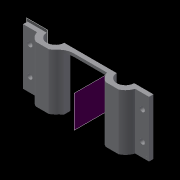
# Autodesk Inventor part: V2 GantryCover
Saved by Autodesk Inventor 2014 (Build 180170000, 170)
## iProperties
Created: 2015-07-08
Part Number: V2 GantryCover
Material: Generic
Document SubType Name: Modeling
Designer: Scott
Density: 1 g/cm^3
Appearance: Default
Author: Scott
Autodesk Inventor part; units mm, degrees
ref_plane "YZ Plane" through (0, 0, 0) normal (1, 0, 0) x (0, 1, 0)
ref_plane "XZ Plane" through (0, 0, 0) normal (0, 1, 0) x (-1, 0, 0)
ref_plane "XY Plane" through (0, 0, 0) normal (0, 0, 1) x (1, 0, 0)
ref_plane "Work Plane1" through (0, 0, 0) normal (0, 0, 1) x (1, 0, 0)
sketch "Sketch1" plane through (0, 0, 0) normal (0, 0, 1) x (1, 0, 0)
  line L0 (-85.1434, -2.54) -> (-85.1434, 45.54) projected
  circle A0 centre (-90.9267, 33.52) radius 2.2225 projected
  circle A1 centre (-90.9267, 9.48) radius 2.2225 projected
  line L1 (-80.2, 45.54) -> (-80.2, -2.54) projected
  line L2 (-80.2, 45.54) -> (-96.71, 45.54) projected
  line L3 (-96.71, 45.54) -> (-96.71, -2.54) projected
  line L4 (-96.71, -2.54) -> (-80.2, -2.54) projected
  line L5 (-20.2, 45.54) -> (-60, 45.54) projected
  circle A2 centre (5.5267, 9.48) radius 2.2225 projected
  circle A3 centre (5.5267, 33.52) radius 2.2225 projected
  line L6 (-5.2, -2.54) -> (-5.2, 45.54) projected
  line L7 (-5.2, -2.54) -> (11.31, -2.54) projected
  line L8 (11.31, 0) -> (11.31, -2.54) projected
  line L9 (11.31, 0) -> (0, 0) projected
  line L10 (0, 0.0064) -> (0, 0) projected
  line L11 (0, 0.0064) -> (11.31, 0.0064) projected
  line L12 (11.31, 0.0064) -> (11.31, 45.54) projected
  line L13 (11.31, 45.54) -> (-5.2, 45.54) projected
  line L14 (-25.4, 27.506) -> (-25.4, 43) projected
  line L15 (-25.4, 27.506) -> (-21.745, 27.506) projected
  line L16 (-21.745, 27.506) -> (-21.745, 3.376) projected
  line L17 (-21.745, 3.376) -> (-25.4, 3.376) projected
  line L18 (-25.4, -2.54) -> (-25.4, 3.376) projected
  line L19 (-25.4, -2.54) -> (-20.2, -2.54) projected
  line L20 (-20.2, 45.54) -> (-20.2, -2.54) projected
  line L21 (-20.2, 45.54) -> (-60, 45.54) projected
  line L22 (-60, 45.54) -> (-60, 43) projected
  line L23 (-60, 43) -> (-25.4, 43) projected
  line L24 (-65.2, -2.54) -> (-65.2, 45.54) projected
  line L25 (-65.2, -2.54) -> (-60, -2.54) projected
  line L26 (-60, 43) -> (-60, -2.54) projected
  line L27 (-60, 45.54) -> (-60, 43) projected
  line L28 (-60, 45.54) -> (-65.2, 45.54) projected
extrude "Extrusion1" add sketch "Sketch1" along normal blind 3.81
sketch "Sketch2" plane through (-96.71, 45.54, 0) normal (0, 1, 0) x (1, 0, 0)
  line L0 (0, 0) -> (16.51, 0) projected
  arc A0 (31.51, 0) -> (16.51, 0) centre (24.01, 0) ccw projected
  arc A1 (16.51, 0) -> (31.51, 0) centre (24.01, 0) ccw
  arc A2 (11.3049, 0) -> (36.7151, 0) centre (24.01, 0) ccw
  line L1 (16.51, 0) -> (11.3049, 0)
  line L2 (31.51, 0) -> (36.7151, 0)
  arc A3 (91.51, 0) -> (76.51, 0) centre (84.01, 0) ccw projected
  arc A4 (76.51, 0) -> (91.51, 0) centre (84.01, 0) ccw
  line L3 (96.71, 0) -> (91.51, 0)
  line L4 (76.51, 0) -> (71.31, 0)
  arc A5 (71.31, 0) -> (96.71, 0) centre (84.01, 0) ccw
  dimension "d3" = 12.7
  constraints: 8 end point, 8 point on circle, 4 centre point, 3 coincident, 3 collinear, 2 concentric, 1 point on line
  measures "d3" radius of A5
extrude "Extrusion2" add sketch "Sketch2" against normal up to surface (48.08 mm away) contours L0 A1 L2 A2 | L3 A5 L4 A4
ref_plane "Work Plane2" through (-42.7, 0, 0) normal (-1, 0, 0) x (0, 0, 1)
sketch "Sketch3" plane through (-42.7, 0, 0) normal (-1, 0, 0) x (0, 0, 1)
  line L0 (12.7051, 45.54) -> (12.7051, -2.54) projected
  line L1 (12.7051, 45.54) -> (11.4351, 45.54)
  line L2 (11.4351, 45.54) -> (11.4351, -2.54)
  line L3 (11.4351, -2.54) -> (12.7051, -2.54)
  line L4 (12.7051, -2.54) -> (12.7051, 45.54)
  point P0 (0, 0)
  dimension "d6" = 1.27
  constraints: 8 end point, 2 parallel, 1 horizontal, 1 perpendicular
  measures "d6" distance of L3.end L2.end
extrude "Extrusion3" cut sketch "Sketch3" along normal mid plane 2540
fillet "Fillet1" radius 12.7 1 edges at (-60.5796, 21.5, 3.81)
body "Solid1"
